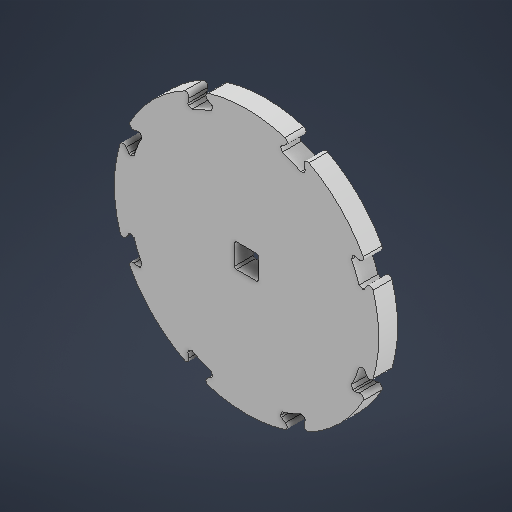
# Autodesk Inventor part: 2in rubberband wheel
Saved by Autodesk Inventor 2025.4 (Build 294407000, 407)
## iProperties
Created: 2026-01-22
Part Number: 2in rubberband wheel
Material: Generic
Document SubType Name: Modeling
Designer: shaun
Density: 1 g/cm^3
Appearance: Default
Author: shaun
Autodesk Inventor part; units mm, degrees
ref_plane "YZ Plane" through (0, 0, 0) normal (1, 0, 0) x (0, 1, 0)
ref_plane "XZ Plane" through (0, 0, 0) normal (0, 1, 0) x (-1, 0, 0)
ref_plane "XY Plane" through (0, 0, 0) normal (0, 0, 1) x (1, 0, 0)
sketch "Sketch1" plane through (0, 0, 0) normal (0, 0, 1) x (1, 0, 0)
  circle A0 centre (0, 0) radius 31.75
  line L0 (-2.7178, -3.2258) -> (2.7178, -3.2258)
  line L1 (3.2258, -2.7178) -> (3.2258, 2.7178)
  line L2 (2.7178, 3.2258) -> (-2.7178, 3.2258)
  line L3 (-3.2258, 2.7178) -> (-3.2258, -2.7178)
  line L4 (-3.2258, -3.2258) -> (3.2258, 3.2258) construction
  line L5 (3.2258, -3.2258) -> (-3.2258, 3.2258) construction
  arc A1 (-2.7178, 3.2258) -> (-3.2258, 2.7178) centre (-2.7178, 2.7178) ccw
  arc A2 (3.2258, 2.7178) -> (2.7178, 3.2258) centre (2.7178, 2.7178) ccw
  arc A3 (2.7178, -3.2258) -> (3.2258, -2.7178) centre (2.7178, -2.7178) ccw
  arc A4 (-3.2258, -2.7178) -> (-2.7178, -3.2258) centre (-2.7178, -2.7178) ccw
  line L6 (-12.1502, 29.3332) -> (-12.1502, -29.3332) construction
  line L7 (12.1502, 29.3332) -> (12.1502, -29.3332) construction
  line L8 (29.3332, 12.1502) -> (-29.3332, 12.1502) construction
  line L9 (-29.3332, -12.1502) -> (29.3332, -12.1502) construction
  line L10 (12.1502, 29.3332) -> (29.3332, 12.1502) construction
  line L11 (29.3332, 12.1502) -> (29.3332, -12.1502) construction
  line L12 (29.3332, -12.1502) -> (12.1502, -29.3332) construction
  line L13 (12.1502, -29.3332) -> (-12.1502, -29.3332) construction
  line L14 (-12.1502, -29.3332) -> (-29.3332, -12.1502) construction
  line L15 (-29.3332, -12.1502) -> (-29.3332, 12.1502) construction
  line L16 (-29.3332, 12.1502) -> (-12.1502, 29.3332) construction
  line L17 (-12.1502, 29.3332) -> (12.1502, 29.3332) construction
  circle A5 centre (0, 0) radius 35.56
  line L18 (0, 0) -> (13.6082, 32.8532) construction
  line L19 (10.3158, 34.0308) -> (8.8498, 30.4917)
  line L20 (15.3031, 27.8186) -> (16.7691, 31.3578)
  arc A6 (9.6387, 32.3961) -> (10.3158, 34.0308) centre (10.0579, 33.1801) ccw
  arc A7 (16.7691, 31.3578) -> (16.092, 29.7231) centre (16.3499, 30.5739) ccw
  point P0 (16.092, 29.7231)
  dimension "d4" = 63.5
  dimension "d2" = 0.508
  dimension "d3" = 6.4516
  dimension "d9" = 6.985
  dimension "d10" = 3.81
  dimension "d11" = 0.889
  constraints: 42 end point, 15 point on circle, 10 point on line, 9 tangent, 7 centre point, 4 coincident, 4 parallel, 3 equal radius, 3 horizontal, 3 perpendicular, 2 midpoint, 2 symmetric about line, 2 vertical, 31 other
  measures "d2" radius of A1
  measures "d3" distance between parallel lines of L1 L3
  measures "d9" distance between parallel lines of L20 L19
  measures "d11" radius of A6
extrude "Extrusion1" add sketch "Sketch1" along normal blind 5.08
extrude "Extrusion2" cut sketch "Sketch1" along normal through all contours A0 L19 A6 A5 A7 L20
chamfer "Chamfer2" distance 0.7937 angle 45 4 edges at (9.6387, 32.3961, 2.54) (8.8498, 30.4917, 2.54) (15.3031, 27.8186, 2.54) (16.092, 29.7231, 2.54)
pattern_circular "Circular Pattern1" count 8 over 360 about axis through (0, 0, 0) along (0, 0, 1) of "Extrusion2", "Chamfer2"
body "Solid1"
